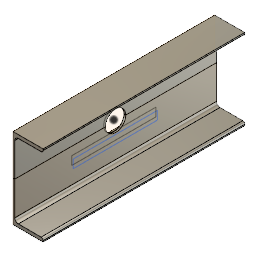
(25;;5@ 24_ (Autodesk Fusion 360 design; units mm, degrees)
Autodesk Fusion 360 part; units mm, degrees
sketch "Sketch1" plane through (0, 0, 0) normal (0, 0, 1) x (1, 0, 0)
  line L0 (0, 0) -> (0, 120)
  line L1 (0, 120) -> (90, 120)
  line L2 (5.6, 99.5) -> (5.6, 0)
  line L3 (90, 116) -> (90, 120)
  line L4 (0, 0) -> (5.6, 0)
  line L5 (16.1, 110) -> (84, 110)
  arc A0 (16.1, 110) -> (5.6, 99.5) centre (16.1, 99.5) ccw
  arc A1 (84, 110) -> (90, 116) centre (84, 116) ccw
  line L6 (0, -120) -> (90, -120)
  arc A2 (5.6, -99.5) -> (16.1, -110) centre (16.1, -99.5) ccw
  line L7 (90, -116) -> (90, -120)
  arc A3 (90, -116) -> (84, -110) centre (84, -116) ccw
  line L8 (16.1, -110) -> (84, -110)
  line L9 (0, 0) -> (0, -120)
  line L10 (5.6, -99.5) -> (5.6, 0)
  dimension "d3" = 120
  dimension "d4" = 90
  dimension "d5" = 5.6
  dimension "d8" = 10.5
  dimension "d9" = 6
  dimension "d10" = 10
  measures "d5" distance of L0.start
  measures "d8" radius of A0
  measures "d9" radius of A1
  measures "d10" distance of L1 L5
extrude "Extrude1" add sketch "Sketch1" along normal blind 600 makes body 1
sketch "Sketch2" plane through (0, 0, 0) normal (-1, 0, 0) x (0, 0, 1)
  line L0 (0, 120) -> (0, -120)
  line L1 (0, -120) -> (600, -120)
  line L2 (600, -120) -> (600, 120)
  line L3 (600, 120) -> (0, 120)
  circle A0 centre (300, 0) radius 30
  line L4 (175, -30) -> (425, -30)
  line L5 (425, -30) -> (425, -55)
  line L6 (425, -55) -> (175, -55)
  line L7 (175, -55) -> (175, -30)
  dimension "d13" = 60
  dimension "d14" = 300
  dimension "d15" = 120
  dimension "d22" = 250
  dimension "d23" = 25
  dimension "d24" = 125
  dimension "d25" = 30
  measures "d13" diameter of A0
  measures "d15" distance of L3 origin
  measures "d22" distance of L5 L7
  measures "d23" distance of L4 L6
  measures "d24" distance of origin L5
  measures "d25" distance of origin L4
extrude "Extrude3" add sketch "Sketch2" along normal blind 5.6 contours L4 L5 L6 L7 bodies 1
extrude "Extrude2" cut sketch "Sketch2" along normal through all and the other way blind 200 contours A0 bodies 1
split "Split1" by plane through (0, 0, 0) normal (0, 1, 0) bodies 1 makes body 2 at (0, 42.9476, 90.4443)
sketch "Sketch3" plane through (5.6, 0, 0) normal (1, 0, 0) x (0, 0, -1)
  line L0 (-330, 0) -> (-600, 0)
  line L1 (-600, 0) -> (-600, -99.5)
  line L2 (-600, -99.5) -> (0, -99.5)
  line L3 (0, -99.5) -> (0, 0)
  line L4 (0, 0) -> (-270, 0)
  arc A0 (-330, 0) -> (-270, 0) centre (-300, 0) ccw
  line L5 (-426.0439, -34.9914) -> (-176.0439, -34.9914)
  line L6 (-176.0439, -34.9914) -> (-176.0439, -59.9914)
  line L7 (-176.0439, -59.9914) -> (-426.0439, -59.9914)
  line L8 (-426.0439, -59.9914) -> (-426.0439, -34.9914)
  dimension "d20" = 250
  dimension "d21" = 25
  measures "d20" distance of L3.end
equation "d3 = ( 240 / 2 ) * 1 mm"
